Autodesk Fusion 360 part; units mm, degrees
(part 10 of 11)
  spline S28 degree 5 poles (78.2014, 31.4697) (78.2336, 31.4825) (78.2976, 31.5088) (78.3926, 31.5505) (78.5172, 31.6105) (78.6702, 31.6914) (78.8212, 31.7765) (78.9711, 31.8642) (79.1202, 31.9533) (79.269, 32.0433) (79.4172, 32.1344) (79.5647, 32.2267) (79.7114, 32.3207) (79.8571, 32.4168) (80.0017, 32.5149) (80.1454, 32.6148) (80.2882, 32.7163) (80.4303, 32.8191) (80.5718, 32.923) (80.7127, 33.028) (80.853, 33.134) (80.9927, 33.2412) (81.1316, 33.3495) (81.2699, 33.4591) (81.4075, 33.5698) (81.5445, 33.6817) (81.6808, 33.7946) (81.8165, 33.9086) (81.9516, 34.0235) (82.0861, 34.1394) (82.22, 34.2562) (82.3534, 34.374) (82.4862, 34.4927) (82.6183, 34.6123) (82.7499, 34.7329) (82.8809, 34.8543) (83.0114, 34.9766) (83.1413, 35.0998) (83.2706, 35.2239) (83.3993, 35.3487) (83.5276, 35.4744) (83.6552, 35.6009) (83.7824, 35.7282) (83.909, 35.8563) (84.035, 35.9852) (84.1605, 36.1148) (84.2855, 36.2452) (84.4099, 36.3764) (84.5338, 36.5083) (84.6572, 36.641) (84.78, 36.7743) (84.9023, 36.9084) (85.0241, 37.0433) (85.1454, 37.1788) (85.2662, 37.315) (85.3864, 37.4519) (85.5062, 37.5895) (85.6254, 37.7277) (85.7441, 37.8667) (85.8623, 38.0063) (85.9799, 38.1465) (86.0971, 38.2874) (86.2138, 38.429) (86.3299, 38.5712) (86.4456, 38.714) (86.5607, 38.8574) (86.6754, 39.0015) (86.7895, 39.1462) (86.9032, 39.2915) (87.0163, 39.4374) (87.1289, 39.5839) (87.2186, 39.7016) (87.2857, 39.7901) (87.3303, 39.8493) (87.3526, 39.8789) knots 0 0 0 0 0 0 0.01428571 0.02857143 0.04285714 0.05714286 0.07142857 0.08571429 0.1 0.11428571 0.12857143 0.14285714 0.15714286 0.17142857 0.18571429 0.2 0.21428571 0.22857143 0.24285714 0.25714286 0.27142857 0.28571429 0.3 0.31428571 0.32857143 0.34285714 0.35714286 0.37142857 0.38571429 0.4 0.41428571 0.42857143 0.44285714 0.45714286 0.47142857 0.48571429 0.5 0.51428571 0.52857143 0.54285714 0.55714286 0.57142857 0.58571429 0.6 0.61428571 0.62857143 0.64285714 0.65714286 0.67142857 0.68571429 0.7 0.71428571 0.72857143 0.74285714 0.75714286 0.77142857 0.78571429 0.8 0.81428571 0.82857143 0.84285714 0.85714286 0.87142857 0.88571429 0.9 0.91428571 0.92857143 0.94285714 0.95714286 0.97142857 0.98571429 1 1 1 1 1 1
  arc A62 (87.3526, 39.8789) -> (85.3387, 44.0607) centre (0.5538, 0.6546) ccw
  spline S29 degree 5 poles (73.0585, 42.1491) (73.0885, 42.1663) (73.149, 42.1999) (73.2409, 42.2481) (73.3654, 42.3082) (73.5241, 42.3774) (73.6848, 42.4424) (73.8468, 42.5049) (74.0095, 42.5659) (74.1726, 42.6261) (74.3362, 42.6852) (74.5003, 42.743) (74.6653, 42.799) (74.8313, 42.853) (74.9981, 42.9049) (75.1658, 42.955) (75.3342, 43.0033) (75.5032, 43.0504) (75.6727, 43.0962) (75.8426, 43.1409) (76.013, 43.1845) (76.1838, 43.2269) (76.3552, 43.268) (76.527, 43.3078) (76.6994, 43.3463) (76.8722, 43.3837) (77.0455, 43.4198) (77.2192, 43.4548) (77.3933, 43.4888) (77.5678, 43.5217) (77.7426, 43.5536) (77.9179, 43.5844) (78.0934, 43.6142) (78.2694, 43.643) (78.4457, 43.6707) (78.6223, 43.6974) (78.7993, 43.7231) (78.9766, 43.7478) (79.1542, 43.7716) (79.3321, 43.7945) (79.5103, 43.8163) (79.6888, 43.8373) (79.8676, 43.8573) (80.0467, 43.8764) (80.226, 43.8946) (80.4056, 43.9119) (80.5855, 43.9283) (80.7656, 43.9438) (80.946, 43.9584) (81.1267, 43.9722) (81.3075, 43.985) (81.4886, 43.9971) (81.67, 44.0083) (81.8515, 44.0186) (82.0333, 44.0281) (82.2153, 44.0367) (82.3976, 44.0445) (82.58, 44.0515) (82.7626, 44.0577) (82.9454, 44.0631) (83.1285, 44.0677) (83.3117, 44.0714) (83.4951, 44.0744) (83.6787, 44.0765) (83.8625, 44.0779) (84.0464, 44.0785) (84.2305, 44.0783) (84.4148, 44.0773) (84.5993, 44.0756) (84.7839, 44.0731) (84.9686, 44.0698) (85.1166, 44.0665) (85.2276, 44.0638) (85.3017, 44.0618) (85.3387, 44.0607) knots 0 0 0 0 0 0 0.01428571 0.02857143 0.04285714 0.05714286 0.07142857 0.08571429 0.1 0.11428571 0.12857143 0.14285714 0.15714286 0.17142857 0.18571429 0.2 0.21428571 0.22857143 0.24285714 0.25714286 0.27142857 0.28571429 0.3 0.31428571 0.32857143 0.34285714 0.35714286 0.37142857 0.38571429 0.4 0.41428571 0.42857143 0.44285714 0.45714286 0.47142857 0.48571429 0.5 0.51428571 0.52857143 0.54285714 0.55714286 0.57142857 0.58571429 0.6 0.61428571 0.62857143 0.64285714 0.65714286 0.67142857 0.68571429 0.7 0.71428571 0.72857143 0.74285714 0.75714286 0.77142857 0.78571429 0.8 0.81428571 0.82857143 0.84285714 0.85714286 0.87142857 0.88571429 0.9 0.91428571 0.92857143 0.94285714 0.95714286 0.97142857 0.98571429 1 1 1 1 1 1
  line L29 (73.0585, 42.1491) -> (71.7614, 41.4071)
  arc A63 (70.6822, 41.6951) -> (71.7614, 41.4071) centre (71.3673, 42.096) ccw
  arc A64 (70.6822, 41.6951) -> (67.9576, 46.0313) centre (0.5538, 0.6546) ccw
  arc A65 (68.1663, 47.1287) -> (67.9576, 46.0313) centre (68.616, 46.4746) ccw
  line L30 (68.1663, 47.1287) -> (69.3976, 47.9753)
  spline S30 degree 5 poles (69.3976, 47.9753) (69.4262, 47.9949) (69.4827, 48.0348) (69.566, 48.0966) (69.6741, 48.1828) (69.8053, 48.2957) (69.9336, 48.4123) (70.0602, 48.5312) (70.1858, 48.6512) (70.3108, 48.7721) (70.435, 48.8938) (70.5583, 49.0167) (70.6804, 49.141) (70.801, 49.2671) (70.9202, 49.3949) (71.038, 49.5243) (71.1547, 49.655) (71.2704, 49.7869) (71.3852, 49.9197) (71.4992, 50.0534) (71.6124, 50.1879) (71.7247, 50.3235) (71.8361, 50.46) (71.9465, 50.5976) (72.0561, 50.7362) (72.1647, 50.8757) (72.2724, 51.0162) (72.3794, 51.1575) (72.4855, 51.2996) (72.5909, 51.4425) (72.6954, 51.5862) (72.7992, 51.7307) (72.9023, 51.8759) (73.0045, 52.022) (73.106, 52.1688) (73.2067, 52.3164) (73.3066, 52.4646) (73.4058, 52.6136) (73.5043, 52.7633) (73.6021, 52.9137) (73.6991, 53.0648) (73.7954, 53.2165) (73.8911, 53.3689) (73.986, 53.522) (74.0802, 53.6757) (74.1737, 53.83) (74.2665, 53.9849) (74.3586, 54.1405) (74.45, 54.2967) (74.5408, 54.4535) (74.6309, 54.6108) (74.7203, 54.7688) (74.8091, 54.9273) (74.8972, 55.0864) (74.9846, 55.2461) (75.0713, 55.4063) (75.1575, 55.5671) (75.2429, 55.7284) (75.3277, 55.8903) (75.4119, 56.0527) (75.4954, 56.2156) (75.5783, 56.3791) (75.6605, 56.543) (75.7421, 56.7075) (75.8231, 56.8725) (75.9034, 57.0379) (75.9831, 57.2039) (76.0622, 57.3704) (76.1407, 57.5373) (76.2185, 57.7047) (76.2957, 57.8726) (76.357, 58.0073) (76.4027, 58.1086) (76.433, 58.1761) (76.4482, 58.21) knots 0 0 0 0 0 0 0.01428571 0.02857143 0.04285714 0.05714286 0.07142857 0.08571429 0.1 0.11428571 0.12857143 0.14285714 0.15714286 0.17142857 0.18571429 0.2 0.21428571 0.22857143 0.24285714 0.25714286 0.27142857 0.28571429 0.3 0.31428571 0.32857143 0.34285714 0.35714286 0.37142857 0.38571429 0.4 0.41428571 0.42857143 0.44285714 0.45714286 0.47142857 0.48571429 0.5 0.51428571 0.52857143 0.54285714 0.55714286 0.57142857 0.58571429 0.6 0.61428571 0.62857143 0.64285714 0.65714286 0.67142857 0.68571429 0.7 0.71428571 0.72857143 0.74285714 0.75714286 0.77142857 0.78571429 0.8 0.81428571 0.82857143 0.84285714 0.85714286 0.87142857 0.88571429 0.9 0.91428571 0.92857143 0.94285714 0.95714286 0.97142857 0.98571429 1 1 1 1 1 1
  arc A66 (76.4482, 58.21) -> (73.5542, 61.8389) centre (0.5538, 0.6546) ccw
  spline S31 degree 5 poles (62.0072, 57.2425) (62.0327, 57.266) (62.0842, 57.3122) (62.163, 57.3797) (62.2711, 57.4659) (62.4104, 57.5687) (62.5526, 57.6679) (62.6966, 57.7648) (62.8416, 57.8605) (62.9873, 57.9555) (63.1336, 58.0495) (63.2808, 58.1424) (63.4292, 58.2337) (63.579, 58.3233) (63.7301, 58.411) (63.8824, 58.4971) (64.0358, 58.5818) (64.1901, 58.6652) (64.3452, 58.7476) (64.5009, 58.829) (64.6573, 58.9094) (64.8144, 58.9887) (64.9723, 59.067) (65.131, 59.144) (65.2905, 59.22) (65.4507, 59.2948) (65.6116, 59.3686) (65.7731, 59.4414) (65.9353, 59.5133) (66.0981, 59.5842) (66.2614, 59.6542) (66.4254, 59.7232) (66.5899, 59.7913) (66.7551, 59.8585) (66.9208, 59.9248) (67.0871, 59.9901) (67.2539, 60.0545) (67.4212, 60.1181) (67.5891, 60.1808) (67.7575, 60.2427) (67.9263, 60.3037) (68.0957, 60.3638) (68.2655, 60.4231) (68.4359, 60.4816) (68.6067, 60.5392) (68.7779, 60.596) (68.9497, 60.652) (69.1218, 60.7072) (69.2944, 60.7616) (69.4675, 60.8152) (69.6409, 60.8681) (69.8148, 60.9201) (69.9891, 60.9713) (70.1639, 61.0218) (70.339, 61.0715) (70.5145, 61.1204) (70.6904, 61.1686) (70.8667, 61.216) (71.0434, 61.2627) (71.2204, 61.3086) (71.3978, 61.3538) (71.5756, 61.3982) (71.7538, 61.4419) (71.9323, 61.4849) (72.1112, 61.5271) (72.2904, 61.5686) (72.4699, 61.6094) (72.6498, 61.6494) (72.83, 61.6888) (73.0105, 61.7274) (73.1914, 61.7653) (73.3364, 61.7951) (73.4452, 61.8171) (73.5179, 61.8316) (73.5542, 61.8389) knots 0 0 0 0 0 0 0.01428571 0.02857143 0.04285714 0.05714286 0.07142857 0.08571429 0.1 0.11428571 0.12857143 0.14285714 0.15714286 0.17142857 0.18571429 0.2 0.21428571 0.22857143 0.24285714 0.25714286 0.27142857 0.28571429 0.3 0.31428571 0.32857143 0.34285714 0.35714286 0.37142857 0.38571429 0.4 0.41428571 0.42857143 0.44285714 0.45714286 0.47142857 0.48571429 0.5 0.51428571 0.52857143 0.54285714 0.55714286 0.57142857 0.58571429 0.6 0.61428571 0.62857143 0.64285714 0.65714286 0.67142857 0.68571429 0.7 0.71428571 0.72857143 0.74285714 0.75714286 0.77142857 0.78571429 0.8 0.81428571 0.82857143 0.84285714 0.85714286 0.87142857 0.88571429 0.9 0.91428571 0.92857143 0.94285714 0.95714286 0.97142857 0.98571429 1 1 1 1 1 1
  line L31 (62.0072, 57.2425) -> (60.9079, 56.2305)
  arc A67 (59.7916, 56.2712) -> (60.9079, 56.2305) centre (60.3703, 56.8145) ccw
  arc A68 (59.7916, 56.2712) -> (56.1704, 59.8924) centre (0.5538, 0.6546) ccw
  arc A69 (56.1297, 61.0086) -> (56.1704, 59.8924) centre (56.7137, 60.4711) ccw
  line L32 (56.1297, 61.0086) -> (57.1417, 62.108)
  spline S32 degree 5 poles (57.1417, 62.108) (57.1652, 62.1335) (57.2114, 62.185) (57.2789, 62.2638) (57.3651, 62.3719) (57.4679, 62.5112) (57.5671, 62.6534) (57.664, 62.7974) (57.7597, 62.9424) (57.8547, 63.0881) (57.9487, 63.2344) (58.0416, 63.3816) (58.1329, 63.53) (58.2225, 63.6797) (58.3102, 63.8309) (58.3963, 63.9832) (58.481, 64.1366) (58.5644, 64.2909) (58.6468, 64.4459) (58.7282, 64.6017) (58.8086, 64.7581) (58.8879, 64.9152) (58.9662, 65.0731) (59.0432, 65.2318) (59.1192, 65.3913) (59.194, 65.5515) (59.2678, 65.7124) (59.3406, 65.8739) (59.4125, 66.0361) (59.4834, 66.1989) (59.5534, 66.3622) (59.6224, 66.5262) (59.6905, 66.6907) (59.7577, 66.8559) (59.824, 67.0216) (59.8893, 67.1879) (59.9537, 67.3547) (60.0173, 67.522) (60.08, 67.6899) (60.1419, 67.8583) (60.2029, 68.0271) (60.263, 68.1965) (60.3223, 68.3663) (60.3808, 68.5367) (60.4384, 68.7075) (60.4952, 68.8787) (60.5512, 69.0505) (60.6064, 69.2226) (60.6608, 69.3952) (60.7144, 69.5683) (60.7673, 69.7417) (60.8193, 69.9156) (60.8705, 70.0899) (60.921, 70.2647) (60.9707, 70.4398) (61.0196, 70.6153) (61.0678, 70.7912) (61.1152, 70.9675) (61.1619, 71.1442) (61.2078, 71.3212) (61.253, 71.4986) (61.2974, 71.6764) (61.3411, 71.8546) (61.3841, 72.0331) (61.4263, 72.212) (61.4678, 72.3912) (61.5086, 72.5707) (61.5486, 72.7506) (61.588, 72.9308) (61.6266, 73.1113) (61.6645, 73.2922) (61.6943, 73.4372) (61.7163, 73.546) (61.7308, 73.6187) (61.7381, 73.655) knots 0 0 0 0 0 0 0.01428571 0.02857143 0.04285714 0.05714286 0.07142857 0.08571429 0.1 0.11428571 0.12857143 0.14285714 0.15714286 0.17142857 0.18571429 0.2 0.21428571 0.22857143 0.24285714 0.25714286 0.27142857 0.28571429 0.3 0.31428571 0.32857143 0.34285714 0.35714286 0.37142857 0.38571429 0.4 0.41428571 0.42857143 0.44285714 0.45714286 0.47142857 0.48571429 0.5 0.51428571 0.52857143 0.54285714 0.55714286 0.57142857 0.58571429 0.6 0.61428571 0.62857143 0.64285714 0.65714286 0.67142857 0.68571429 0.7 0.71428571 0.72857143 0.74285714 0.75714286 0.77142857 0.78571429 0.8 0.81428571 0.82857143 0.84285714 0.85714286 0.87142857 0.88571429 0.9 0.91428571 0.92857143 0.94285714 0.95714286 0.97142857 0.98571429 1 1 1 1 1 1
  arc A70 (61.7381, 73.655) -> (58.1092, 76.549) centre (0.5538, 0.6546) ccw
  spline S33 degree 5 poles (47.8745, 69.4984) (47.8941, 69.527) (47.934, 69.5835) (47.9958, 69.6668) (48.082, 69.7749) (48.1949, 69.9061) (48.3115, 70.0344) (48.4304, 70.161) (48.5504, 70.2866) (48.6713, 70.4116) (48.793, 70.5358) (48.9159, 70.6591) (49.0402, 70.7812) (49.1663, 70.9018) (49.2941, 71.021) (49.4235, 71.1388) (49.5542, 71.2555) (49.6861, 71.3712) (49.8189, 71.486) (49.9526, 71.6) (50.0871, 71.7132) (50.2227, 71.8255) (50.3592, 71.9369) (50.4968, 72.0473) (50.6354, 72.1569) (50.7749, 72.2655) (50.9154, 72.3732) (51.0567, 72.4802) (51.1988, 72.5863) (51.3417, 72.6917) (51.4854, 72.7962) (51.6299, 72.9) (51.7751, 73.0031) (51.9212, 73.1053) (52.068, 73.2068) (52.2156, 73.3075) (52.3638, 73.4074) (52.5129, 73.5066) (52.6626, 73.6051) (52.8129, 73.7029) (52.964, 73.7999) (53.1157, 73.8962) (53.2681, 73.9919) (53.4212, 74.0868) (53.5749, 74.181) (53.7292, 74.2745) (53.8842, 74.3673) (54.0397, 74.4594) (54.1959, 74.5508) (54.3527, 74.6416) (54.51, 74.7317) (54.668, 74.8211) (54.8265, 74.9099) (54.9856, 74.998) (55.1453, 75.0854) (55.3055, 75.1721) (55.4663, 75.2583) (55.6276, 75.3437) (55.7895, 75.4285) (55.9519, 75.5127) (56.1148, 75.5962) (56.2783, 75.6791) (56.4422, 75.7613) (56.6067, 75.8429) (56.7717, 75.9239) (56.9371, 76.0042) (57.1031, 76.0839) (57.2696, 76.163) (57.4365, 76.2415) (57.6039, 76.3193) (57.7718, 76.3965) (57.9065, 76.4578) (58.0078, 76.5035) (58.0753, 76.5338) (58.1092, 76.549) knots 0 0 0 0 0 0 0.01428571 0.02857143 0.04285714 0.05714286 0.07142857 0.08571429 0.1 0.11428571 0.12857143 0.14285714 0.15714286 0.17142857 0.18571429 0.2 0.21428571 0.22857143 0.24285714 0.25714286 0.27142857 0.28571429 0.3 0.31428571 0.32857143 0.34285714 0.35714286 0.37142857 0.38571429 0.4 0.41428571 0.42857143 0.44285714 0.45714286 0.47142857 0.48571429 0.5 0.51428571 0.52857143 0.54285714 0.55714286 0.57142857 0.58571429 0.6 0.61428571 0.62857143 0.64285714 0.65714286 0.67142857 0.68571429 0.7 0.71428571 0.72857143 0.74285714 0.75714286 0.77142857 0.78571429 0.8 0.81428571 0.82857143 0.84285714 0.85714286 0.87142857 0.88571429 0.9 0.91428571 0.92857143 0.94285714 0.95714286 0.97142857 0.98571429 1 1 1 1 1 1
  line L33 (47.8745, 69.4984) -> (47.0279, 68.2671)
  arc A71 (45.9305, 68.0584) -> (47.0279, 68.2671) centre (46.3738, 68.7168) ccw
  arc A72 (45.9305, 68.0584) -> (41.5943, 70.783) centre (0.5538, 0.6546) ccw
  arc A73 (41.3063, 71.8622) -> (41.5943, 70.783) centre (41.9952, 71.4681) ccw
  line L34 (41.3063, 71.8622) -> (42.0483, 73.1593)
  spline S34 degree 5 poles (42.0483, 73.1593) (42.0655, 73.1893) (42.0991, 73.2498) (42.1473, 73.3417) (42.2074, 73.4662) (42.2766, 73.6249) (42.3416, 73.7856) (42.4041, 73.9476) (42.4651, 74.1103) (42.5253, 74.2734) (42.5844, 74.437) (42.6422, 74.6011) (42.6982, 74.7661) (42.7522, 74.9321) (42.8041, 75.0989) (42.8542, 75.2666) (42.9025, 75.435) (42.9496, 75.604) (42.9954, 75.7735) (43.0401, 75.9434) (43.0837, 76.1138) (43.1261, 76.2846) (43.1672, 76.456) (43.207, 76.6278) (43.2456, 76.8002) (43.2829, 76.973) (43.319, 77.1463) (43.354, 77.32) (43.388, 77.4941) (43.4209, 77.6686) (43.4528, 77.8434) (43.4836, 78.0187) (43.5134, 78.1942) (43.5422, 78.3702) (43.5699, 78.5465) (43.5966, 78.7231) (43.6223, 78.9001) (43.6471, 79.0774) (43.6708, 79.255) (43.6937, 79.4329) (43.7155, 79.6111) (43.7365, 79.7896) (43.7565, 79.9684) (43.7756, 80.1475) (43.7938, 80.3268) (43.8111, 80.5064) (43.8275, 80.6863) (43.843, 80.8664) (43.8576, 81.0468) (43.8714, 81.2275) (43.8842, 81.4083) (43.8963, 81.5894) (43.9075, 81.7708) (43.9178, 81.9523) (43.9273, 82.1341) (43.9359, 82.3161) (43.9437, 82.4984) (43.9507, 82.6808) (43.9569, 82.8634) (43.9623, 83.0462) (43.9669, 83.2293) (43.9706, 83.4125) (43.9736, 83.5959) (43.9757, 83.7795) (43.9771, 83.9633) (43.9777, 84.1472) (43.9775, 84.3313) (43.9765, 84.5156) (43.9748, 84.7001) (43.9723, 84.8847) (43.969, 85.0694) (43.9657, 85.2174) (43.963, 85.3284) (43.961, 85.4025) (43.9599, 85.4395) knots 0 0 0 0 0 0 0.01428571 0.02857143 0.04285714 0.05714286 0.07142857 0.08571429 0.1 0.11428571 0.12857143 0.14285714 0.15714286 0.17142857 0.18571429 0.2 0.21428571 0.22857143 0.24285714 0.25714286 0.27142857 0.28571429 0.3 0.31428571 0.32857143 0.34285714 0.35714286 0.37142857 0.38571429 0.4 0.41428571 0.42857143 0.44285714 0.45714286 0.47142857 0.48571429 0.5 0.51428571 0.52857143 0.54285714 0.55714286 0.57142857 0.58571429 0.6 0.61428571 0.62857143 0.64285714 0.65714286 0.67142857 0.68571429 0.7 0.71428571 0.72857143 0.74285714 0.75714286 0.77142857 0.78571429 0.8 0.81428571 0.82857143 0.84285714 0.85714286 0.87142857 0.88571429 0.9 0.91428571 0.92857143 0.94285714 0.95714286 0.97142857 0.98571429 1 1 1 1 1 1
  arc A74 (43.9599, 85.4395) -> (39.7781, 87.4534) centre (0.5538, 0.6546) ccw
  spline S35 degree 5 poles (31.3689, 78.3022) (31.3817, 78.3344) (31.408, 78.3984) (31.4497, 78.4934) (31.5097, 78.618) (31.5906, 78.771) (31.6757, 78.922) (31.7634, 79.0719) (31.8525, 79.221) (31.9425, 79.3697) (32.0336, 79.518) (32.1259, 79.6655) (32.2199, 79.8122) (32.316, 79.9579) (32.4141, 80.1025) (32.514, 80.2462) (32.6155, 80.389) (32.7183, 80.5311) (32.8222, 80.6726) (32.9272, 80.8135) (33.0332, 80.9538) (33.1404, 81.0935) (33.2487, 81.2324) (33.3583, 81.3707) (33.469, 81.5083) (33.5809, 81.6453) (33.6938, 81.7816) (33.8078, 81.9173) (33.9227, 82.0524) (34.0386, 82.1869) (34.1554, 82.3208) (34.2732, 82.4542) (34.3919, 82.587) (34.5115, 82.7191) (34.6321, 82.8507) (34.7535, 82.9817) (34.8758, 83.1122) (34.999, 83.242) (35.1231, 83.3714) (35.2479, 83.5001) (35.3736, 83.6284) (35.5001, 83.756) (35.6274, 83.8832) (35.7555, 84.0098) (35.8844, 84.1358) (36.014, 84.2613) (36.1444, 84.3863) (36.2756, 84.5107) (36.4075, 84.6346) (36.5402, 84.758) (36.6735, 84.8808) (36.8076, 85.0031) (36.9425, 85.1249) (37.078, 85.2462) (37.2142, 85.367) (37.3511, 85.4872) (37.4887, 85.607) (37.6269, 85.7262) (37.7659, 85.8449) (37.9055, 85.9631) (38.0457, 86.0807) (38.1866, 86.1979) (38.3282, 86.3146) (38.4704, 86.4307) (38.6132, 86.5464) (38.7566, 86.6615) (38.9007, 86.7762) (39.0454, 86.8903) (39.1907, 87.0039) (39.3366, 87.1171) (39.4831, 87.2297) (39.6008, 87.3194) (39.6893, 87.3865) (39.7485, 87.4311) (39.7781, 87.4534) knots 0 0 0 0 0 0 0.01428571 0.02857143 0.04285714 0.05714286 0.07142857 0.08571429 0.1 0.11428571 0.12857143 0.14285714 0.15714286 0.17142857 0.18571429 0.2 0.21428571 0.22857143 0.24285714 0.25714286 0.27142857 0.28571429 0.3 0.31428571 0.32857143 0.34285714 0.35714286 0.37142857 0.38571429 0.4 0.41428571 0.42857143 0.44285714 0.45714286 0.47142857 0.48571429 0.5 0.51428571 0.52857143 0.54285714 0.55714286 0.57142857 0.58571429 0.6 0.61428571 0.62857143 0.64285714 0.65714286 0.67142857 0.68571429 0.7 0.71428571 0.72857143 0.74285714 0.75714286 0.77142857 0.78571429 0.8 0.81428571 0.82857143 0.84285714 0.85714286 0.87142857 0.88571429 0.9 0.91428571 0.92857143 0.94285714 0.95714286 0.97142857 0.98571429 1 1 1 1 1 1
  line L35 (31.3689, 78.3022) -> (30.8175, 76.9134)
  arc A75 (29.7941, 76.4657) -> (30.8175, 76.9134) centre (30.0797, 77.2063) ccw
  arc A76 (29.7941, 76.4657) -> (24.9603, 78.1571) centre (0.5538, 0.6546) ccw
  arc A77 (24.4393, 79.1452) -> (24.9603, 78.1571) centre (25.1987, 78.9142) ccw
  line L36 (24.4393, 79.1452) -> (24.8741, 80.5748)
  spline S36 degree 5 poles (24.8741, 80.5748) (24.8842, 80.6079) (24.9035, 80.6744) (24.9301, 80.7747) (24.9609, 80.9095) (24.9931, 81.0795) (25.0207, 81.2507) (25.0456, 81.4225) (25.0689, 81.5947) (25.0912, 81.7671) (25.1125, 81.9398) (25.1323, 82.1127) (25.1502, 82.286) (25.1659, 82.4598) (25.1794, 82.634) (25.1909, 82.8086) (25.2006, 82.9836) (25.2088, 83.1588) (25.2158, 83.3342) (25.2216, 83.5098) (25.2261, 83.6856) (25.2294, 83.8616) (25.2314, 84.0378) (25.232, 84.2142) (25.2312, 84.3909) (25.2291, 84.5677) (25.2258, 84.7447) (25.2213, 84.9218) (25.2157, 85.0991) (25.209, 85.2765) (25.2011, 85.4541) (25.1922, 85.6318) (25.1822, 85.8096) (25.171, 85.9875) (25.1588, 86.1655) (25.1456, 86.3437) (25.1312, 86.522) (25.1159, 86.7003) (25.0996, 86.8787) (25.0822, 87.0573) (25.0639, 87.2359) (25.0446, 87.4146) (25.0244, 87.5933) (25.0031, 87.7722) (24.981, 87.9511) (24.9578, 88.13) (24.9338, 88.309) (24.9088, 88.4881) (24.8829, 88.6672) (24.8562, 88.8464) (24.8285, 89.0256) (24.7999, 89.2048) (24.7705, 89.3841) (24.7401, 89.5634) (24.7089, 89.7428) (24.6769, 89.9221) (24.6439, 90.1015) (24.6102, 90.2809) (24.5755, 90.4604) (24.5401, 90.6398) (24.5038, 90.8193) (24.4667, 90.9987) (24.4288, 91.1782) (24.39, 91.3576) (24.3505, 91.5371) (24.3101, 91.7166) (24.2689, 91.896) (24.227, 92.0755) (24.1843, 92.2549) (24.1407, 92.4344) (24.0964, 92.6138) (24.0603, 92.7573) (24.0329, 92.8649) (24.0145, 92.9367) (24.0053, 92.9725) knots 0 0 0 0 0 0 0.01428571 0.02857143 0.04285714 0.05714286 0.07142857 0.08571429 0.1 0.11428571 0.12857143 0.14285714 0.15714286 0.17142857 0.18571429 0.2 0.21428571 0.22857143 0.24285714 0.25714286 0.27142857 0.28571429 0.3 0.31428571 0.32857143 0.34285714 0.35714286 0.37142857 0.38571429 0.4 0.41428571 0.42857143 0.44285714 0.45714286 0.47142857 0.48571429 0.5 0.51428571 0.52857143 0.54285714 0.55714286 0.57142857 0.58571429 0.6 0.61428571 0.62857143 0.64285714 0.65714286 0.67142857 0.68571429 0.7 0.71428571 0.72857143 0.74285714 0.75714286 0.77142857 0.78571429 0.8 0.81428571 0.82857143 0.84285714 0.85714286 0.87142857 0.88571429 0.9 0.91428571 0.92857143 0.94285714 0.95714286 0.97142857 0.98571429 1 1 1 1 1 1
  arc A78 (24.0053, 92.9725) -> (19.4801, 94.0054) centre (0.5538, 0.6546) ccw
  spline S37 degree 5 poles (13.3181, 83.2124) (13.3234, 83.2466) (13.3348, 83.3149) (13.3544, 83.4168) (13.3851, 83.5516) (13.4299, 83.7188) (13.4793, 83.8849) (13.5314, 84.0505) (13.5851, 84.2158) (13.6398, 84.3808) (13.6955, 84.5456) (13.7527, 84.71) (13.8118, 84.8739) (13.873, 85.0373) (13.9365, 85.2001) (14.0019, 85.3624) (14.0691, 85.5243) (14.1377, 85.6857) (14.2075, 85.8468) (14.2785, 86.0075) (14.3507, 86.1679) (14.424, 86.3279) (14.4987, 86.4875) (14.5748, 86.6467) (14.6521, 86.8055) (14.7307, 86.9639) (14.8105, 87.1219) (14.8914, 87.2796) (14.9734, 87.4368) (15.0564, 87.5938) (15.1405, 87.7503) (15.2256, 87.9066) (15.3118, 88.0624) (15.399, 88.2179) (15.4873, 88.373) (15.5766, 88.5278) (15.6668, 88.6822) (15.758, 88.8362) (15.8501, 88.9899) (15.9432, 89.1432) (16.0372, 89.2962) (16.1321, 89.4488) (16.2279, 89.6011) (16.3247, 89.753) (16.4223, 89.9045) (16.5207, 90.0557) (16.6201, 90.2066) (16.7203, 90.3571) (16.8213, 90.5072) (16.9232, 90.657) (17.0259, 90.8065) (17.1294, 90.9556) (17.2337, 91.1043) (17.3388, 91.2527) (17.4448, 91.4008) (17.5515, 91.5485) (17.659, 91.6958) (17.7672, 91.8428) (17.8763, 91.9894) (17.9861, 92.1357) (18.0966, 92.2817) (18.2079, 92.4272) (18.32, 92.5725) (18.4327, 92.7174) (18.5462, 92.8619) (18.6605, 93.0061) (18.7754, 93.1499) (18.8911, 93.2934) (19.0075, 93.4365) (19.1245, 93.5793) (19.2423, 93.7217) (19.3371, 93.8353) (19.4084, 93.9204) (19.4562, 93.9771) (19.4801, 94.0054) knots 0 0 0 0 0 0 0.01428571 0.02857143 0.04285714 0.05714286 0.07142857 0.08571429 0.1 0.11428571 0.12857143 0.14285714 0.15714286 0.17142857 0.18571429 0.2 0.21428571 0.22857143 0.24285714 0.25714286 0.27142857 0.28571429 0.3 0.31428571 0.32857143 0.34285714 0.35714286 0.37142857 0.38571429 0.4 0.41428571 0.42857143 0.44285714 0.45714286 0.47142857 0.48571429 0.5 0.51428571 0.52857143 0.54285714 0.55714286 0.57142857 0.58571429 0.6 0.61428571 0.62857143 0.64285714 0.65714286 0.67142857 0.68571429 0.7 0.71428571 0.72857143 0.74285714 0.75714286 0.77142857 0.78571429 0.8 0.81428571 0.82857143 0.84285714 0.85714286 0.87142857 0.88571429 0.9 0.91428571 0.92857143 0.94285714 0.95714286 0.97142857 0.98571429 1 1 1 1 1 1
  line L37 (13.3181, 83.2124) -> (13.0895, 81.7357)
  arc A79 (12.1914, 81.0715) -> (13.0895, 81.7357) centre (12.3051, 81.8571) ccw
  arc A80 (12.1914, 81.0715) -> (7.1025, 81.6449) centre (0.5538, 0.6546) ccw
  arc A81 (6.3747, 82.4923) -> (7.1025, 81.6449) centre (7.1664, 82.4361) ccw
  line L38 (6.3747, 82.4923) -> (6.4805, 83.9828)
  spline S38 degree 5 poles (6.4805, 83.9828) (6.4829, 84.0174) (6.487, 84.0864) (6.4906, 84.1901) (6.4906, 84.3284) (6.4841, 84.5014) (6.473, 84.6744) (6.459, 84.8474) (6.4434, 85.0205) (6.4268, 85.1935) (6.4091, 85.3666) (6.39, 85.5396) (6.3689, 85.7126) (6.3455, 85.8855) (6.3199, 86.0583) (6.2922, 86.2311) (6.2627, 86.4038) (6.2318, 86.5765) (6.1995, 86.7491) (6.1661, 86.9216) (6.1314, 87.094) (6.0955, 87.2663) (6.0582, 87.4385) (6.0195, 87.6106) (5.9794, 87.7827) (5.9381, 87.9546) (5.8954, 88.1264) (5.8516, 88.2981) (5.8067, 88.4697) (5.7607, 88.6412) (5.7135, 88.8125) (5.6653, 88.9838) (5.6159, 89.1549) (5.5655, 89.3259) (5.514, 89.4967) (5.4614, 89.6675) (5.4078, 89.8381) (5.3531, 90.0085) (5.2975, 90.1789) (5.2409, 90.3491) (5.1833, 90.5191) (5.1247, 90.689) (5.0652, 90.8588) (5.0047, 91.0284) (4.9432, 91.1979) (4.8809, 91.3672) (4.8176, 91.5364) (4.7534, 91.7054) (4.6883, 91.8743) (4.6223, 92.043) (4.5555, 92.2116) (4.4877, 92.38) (4.4191, 92.5482) (4.3497, 92.7162) (4.2793, 92.8842) (4.2082, 93.0519) (4.1361, 93.2195) (4.0633, 93.3869) (3.9896, 93.5541) (3.9151, 93.7211) (3.8398, 93.888) (3.7637, 94.0547) (3.6868, 94.2212) (3.6091, 94.3876) (3.5306, 94.5538) (3.4513, 94.7197) (3.3712, 94.8855) (3.2904, 95.0512) (3.2088, 95.2166) (3.1264, 95.3818) (3.0433, 95.5469) (2.9762, 95.6788) (2.9255, 95.7776) (2.8916, 95.8434) (2.8746, 95.8764) knots 0 0 0 0 0 0 0.01428571 0.02857143 0.04285714 0.05714286 0.07142857 0.08571429 0.1 0.11428571 0.12857143 0.14285714 0.15714286 0.17142857 0.18571429 0.2 0.21428571 0.22857143 0.24285714 0.25714286 0.27142857 0.28571429 0.3 0.31428571 0.32857143 0.34285714 0.35714286 0.37142857 0.38571429 0.4 0.41428571 0.42857143 0.44285714 0.45714286 0.47142857 0.48571429 0.5 0.51428571 0.52857143 0.54285714 0.55714286 0.57142857 0.58571429 0.6 0.61428571 0.62857143 0.64285714 0.65714286 0.67142857 0.68571429 0.7 0.71428571 0.72857143 0.74285714 0.75714286 0.77142857 0.78571429 0.8 0.81428571 0.82857143 0.84285714 0.85714286 0.87142857 0.88571429 0.9 0.91428571 0.92857143 0.94285714 0.95714286 0.97142857 0.98571429 1 1 1 1 1 1
  arc A82 (2.8746, 95.8764) -> (-1.7669, 95.8764) centre (0.5538, 0.6546) ccw
  spline S39 degree 5 poles (-5.3728, 83.9828) (-5.3752, 84.0174) (-5.3793, 84.0864) (-5.3829, 84.1901) (-5.3829, 84.3284) (-5.3764, 84.5014) (-5.3653, 84.6744) (-5.3513, 84.8474) (-5.3357, 85.0205) (-5.3191, 85.1935) (-5.3014, 85.3666) (-5.2823, 85.5396) (-5.2612, 85.7126) (-5.2378, 85.8855) (-5.2122, 86.0583) (-5.1845, 86.2311) (-5.155, 86.4038) (-5.1241, 86.5765) (-5.0918, 86.7491) (-5.0584, 86.9216) (-5.0237, 87.094) (-4.9878, 87.2663) (-4.9505, 87.4385) (-4.9118, 87.6106) (-4.8717, 87.7827) (-4.8304, 87.9546) (-4.7877, 88.1264) (-4.7439, 88.2981) (-4.699, 88.4697) (-4.653, 88.6412) (-4.6058, 88.8125) (-4.5576, 88.9838) (-4.5082, 89.1549) (-4.4578, 89.3259) (-4.4063, 89.4967) (-4.3537, 89.6675) (-4.3001, 89.8381) (-4.2454, 90.0085) (-4.1898, 90.1789) (-4.1332, 90.3491) (-4.0756, 90.5191) (-4.017, 90.689) (-3.9575, 90.8588) (-3.897, 91.0284) (-3.8356, 91.1979) (-3.7732, 91.3672) (-3.7099, 91.5364) (-3.6457, 91.7054) (-3.5806, 91.8743) (-3.5147, 92.043) (-3.4478, 92.2116) (-3.3801, 92.38) (-3.3114, 92.5482) (-3.242, 92.7162) (-3.1716, 92.8842) (-3.1005, 93.0519) (-3.0285, 93.2195) (-2.9556, 93.3869) (-2.8819, 93.5541) (-2.8074, 93.7211) (-2.7321, 93.888) (-2.656, 94.0547) (-2.5791, 94.2212) (-2.5014, 94.3876) (-2.4229, 94.5538) (-2.3436, 94.7197) (-2.2636, 94.8855) (-2.1827, 95.0512) (-2.1011, 95.2166) (-2.0188, 95.3818) (-1.9356, 95.5469) (-1.8685, 95.6788) (-1.8179, 95.7776) (-1.7839, 95.8434) (-1.7669, 95.8764) knots 0 0 0 0 0 0 0.01428571 0.02857143 0.04285714 0.05714286 0.07142857 0.08571429 0.1 0.11428571 0.12857143 0.14285714 0.15714286 0.17142857 0.18571429 0.2 0.21428571 0.22857143 0.24285714 0.25714286 0.27142857 0.28571429 0.3 0.31428571 0.32857143 0.34285714 0.35714286 0.37142857 0.38571429 0.4 0.41428571 0.42857143 0.44285714 0.45714286 0.47142857 0.48571429 0.5 0.51428571 0.52857143 0.54285714 0.55714286 0.57142857 0.58571429 0.6 0.61428571 0.62857143 0.64285714 0.65714286 0.67142857 0.68571429 0.7 0.71428571 0.72857143 0.74285714 0.75714286 0.77142857 0.78571429 0.8 0.81428571 0.82857143 0.84285714 0.85714286 0.87142857 0.88571429 0.9 0.91428571 0.92857143 0.94285714 0.95714286 0.97142857 0.98571429 1 1 1 1 1 1
  line L39 (-5.3728, 83.9828) -> (-5.267, 82.4923)
  arc A83 (-5.9948, 81.6449) -> (-5.267, 82.4923) centre (-6.0588, 82.4361) ccw
  arc A84 (-5.9948, 81.6449) -> (-11.0838, 81.0715) centre (0.5538, 0.6546) ccw
  arc A85 (-11.9819, 81.7357) -> (-11.0838, 81.0715) centre (-11.1974, 81.8571) ccw
  line L40 (-11.9819, 81.7357) -> (-12.2104, 83.2124)
  spline S40 degree 5 poles (-12.2104, 83.2124) (-12.2157, 83.2466) (-12.2271, 83.3149) (-12.2467, 83.4168) (-12.2774, 83.5516) (-12.3222, 83.7188) (-12.3716, 83.8849) (-12.4237, 84.0505) (-12.4774, 84.2158) (-12.5321, 84.3808) (-12.5879, 84.5456) (-12.645, 84.71) (-12.7041, 84.8739) (-12.7654, 85.0373) (-12.8288, 85.2001) (-12.8942, 85.3624) (-12.9614, 85.5243) (-13.03, 85.6857) (-13.0998, 85.8468) (-13.1708, 86.0075) (-13.243, 86.1679) (-13.3164, 86.3279) (-13.3911, 86.4875) (-13.4671, 86.6467) (-13.5444, 86.8055) (-13.623, 86.9639) (-13.7028, 87.1219) (-13.7837, 87.2796) (-13.8657, 87.4368) (-13.9487, 87.5938) (-14.0328, 87.7503) (-14.118, 87.9066) (-14.2041, 88.0624) (-14.2914, 88.2179) (-14.3796, 88.373) (-14.4689, 88.5278) (-14.5591, 88.6822) (-14.6503, 88.8362) (-14.7425, 88.9899) (-14.8355, 89.1432) (-14.9295, 89.2962) (-15.0244, 89.4488) (-15.1203, 89.6011) (-15.217, 89.753) (-15.3146, 89.9045) (-15.4131, 90.0557) (-15.5124, 90.2066) (-15.6126, 90.3571) (-15.7136, 90.5072) (-15.8155, 90.657) (-15.9182, 90.8065) (-16.0217, 90.9556) (-16.126, 91.1043) (-16.2312, 91.2527) (-16.3371, 91.4008) (-16.4438, 91.5485) (-16.5513, 91.6958) (-16.6596, 91.8428) (-16.7686, 91.9894) (-16.8784, 92.1357) (-16.9889, 92.2817) (-17.1002, 92.4272) (-17.2123, 92.5725) (-17.3251, 92.7174) (-17.4386, 92.8619) (-17.5528, 93.0061) (-17.6677, 93.1499) (-17.7834, 93.2934) (-17.8998, 93.4365) (-18.0168, 93.5793) (-18.1346, 93.7217) (-18.2294, 93.8353) (-18.3008, 93.9204) (-18.3485, 93.9771) (-18.3724, 94.0054) knots 0 0 0 0 0 0 0.01428571 0.02857143 0.04285714 0.05714286 0.07142857 0.08571429 0.1 0.11428571 0.12857143 0.14285714 0.15714286 0.17142857 0.18571429 0.2 0.21428571 0.22857143 0.24285714 0.25714286 0.27142857 0.28571429 0.3 0.31428571 0.32857143 0.34285714 0.35714286 0.37142857 0.38571429 0.4 0.41428571 0.42857143 0.44285714 0.45714286 0.47142857 0.48571429 0.5 0.51428571 0.52857143 0.54285714 0.55714286 0.57142857 0.58571429 0.6 0.61428571 0.62857143 0.64285714 0.65714286 0.67142857 0.68571429 0.7 0.71428571 0.72857143 0.74285714 0.75714286 0.77142857 0.78571429 0.8 0.81428571 0.82857143 0.84285714 0.85714286 0.87142857 0.88571429 0.9 0.91428571 0.92857143 0.94285714 0.95714286 0.97142857 0.98571429 1 1 1 1 1 1
  arc A86 (-18.3724, 94.0054) -> (-22.8976, 92.9725) centre (0.5538, 0.6546) ccw
  spline S41 degree 5 poles (-23.7664, 80.5748) (-23.7765, 80.6079) (-23.7959, 80.6744) (-23.8224, 80.7747) (-23.8532, 80.9095) (-23.8854, 81.0795) (-23.913, 81.2507) (-23.9379, 81.4225) (-23.9612, 81.5947) (-23.9836, 81.7671) (-24.0048, 81.9398) (-24.0246, 82.1127) (-24.0425, 82.286) (-24.0582, 82.4598) (-24.0717, 82.634) (-24.0832, 82.8086) (-24.0929, 82.9836) (-24.1011, 83.1588) (-24.1081, 83.3342) (-24.1139, 83.5098) (-24.1185, 83.6856) (-24.1218, 83.8616) (-24.1237, 84.0378) (-24.1243, 84.2142) (-24.1235, 84.3909) (-24.1214, 84.5677) (-24.1181, 84.7447) (-24.1136, 84.9218) (-24.108, 85.0991) (-24.1013, 85.2765) (-24.0934, 85.4541) (-24.0845, 85.6318) (-24.0745, 85.8096) (-24.0634, 85.9875) (-24.0512, 86.1655) (-24.0379, 86.3437) (-24.0236, 86.522) (-24.0082, 86.7003) (-23.9919, 86.8787) (-23.9746, 87.0573) (-23.9562, 87.2359) (-23.9369, 87.4146) (-23.9167, 87.5933) (-23.8955, 87.7722) (-23.8733, 87.9511) (-23.8502, 88.13) (-23.8261, 88.309) (-23.8011, 88.4881) (-23.7753, 88.6672) (-23.7485, 88.8464) (-23.7208, 89.0256) (-23.6922, 89.2048) (-23.6628, 89.3841) (-23.6324, 89.5634) (-23.6012, 89.7428) (-23.5692, 89.9221) (-23.5362, 90.1015) (-23.5025, 90.2809) (-23.4679, 90.4604) (-23.4324, 90.6398) (-23.3961, 90.8193) (-23.359, 90.9987) (-23.3211, 91.1782) (-23.2823, 91.3576) (-23.2428, 91.5371) (-23.2024, 91.7166) (-23.1613, 91.896) (-23.1193, 92.0755) (-23.0766, 92.2549) (-23.033, 92.4344) (-22.9887, 92.6138) (-22.9527, 92.7573) (-22.9253, 92.8649) (-22.9068, 92.9367) (-22.8976, 92.9725) knots 0 0 0 0 0 0 0.01428571 0.02857143 0.04285714 0.05714286 0.07142857 0.08571429 0.1 0.11428571 0.12857143 0.14285714 0.15714286 0.17142857 0.18571429 0.2 0.21428571 0.22857143 0.24285714 0.25714286 0.27142857 0.28571429 0.3 0.31428571 0.32857143 0.34285714 0.35714286 0.37142857 0.38571429 0.4 0.41428571 0.42857143 0.44285714 0.45714286 0.47142857 0.48571429 0.5 0.51428571 0.52857143 0.54285714 0.55714286 0.57142857 0.58571429 0.6 0.61428571 0.62857143 0.64285714 0.65714286 0.67142857 0.68571429 0.7 0.71428571 0.72857143 0.74285714 0.75714286 0.77142857 0.78571429 0.8 0.81428571 0.82857143 0.84285714 0.85714286 0.87142857 0.88571429 0.9 0.91428571 0.92857143 0.94285714 0.95714286 0.97142857 0.98571429 1 1 1 1 1 1
  line L41 (-23.7664, 80.5748) -> (-23.3316, 79.1452)
  arc A87 (-23.8526, 78.1571) -> (-23.3316, 79.1452) centre (-24.091, 78.9142) ccw
  arc A88 (-23.8526, 78.1571) -> (-28.6864, 76.4657) centre (0.5538, 0.6546) ccw
  arc A89 (-29.7098, 76.9134) -> (-28.6864, 76.4657) centre (-28.9721, 77.2063) ccw
  line L42 (-29.7098, 76.9134) -> (-30.2612, 78.3022)
  spline S42 degree 5 poles (-30.2612, 78.3022) (-30.274, 78.3344) (-30.3003, 78.3984) (-30.342, 78.4934) (-30.402, 78.618) (-30.4829, 78.771) (-30.568, 78.922) (-30.6557, 79.0719) (-30.7448, 79.221) (-30.8349, 79.3697) (-30.9259, 79.518) (-31.0182, 79.6655) (-31.1123, 79.8122) (-31.2083, 79.9579) (-31.3064, 80.1025) (-31.4063, 80.2462) (-31.5078, 80.389) (-31.6106, 80.5311) (-31.7145, 80.6726) (-31.8195, 80.8135) (-31.9255, 80.9538) (-32.0327, 81.0935) (-32.141, 81.2324) (-32.2506, 81.3707) (-32.3613, 81.5083) (-32.4732, 81.6453) (-32.5861, 81.7816) (-32.7001, 81.9173) (-32.815, 82.0524) (-32.9309, 82.1869) (-33.0477, 82.3208) (-33.1655, 82.4542) (-33.2842, 82.587) (-33.4038, 82.7191) (-33.5244, 82.8507) (-33.6458, 82.9817) (-33.7682, 83.1122) (-33.8914, 83.242) (-34.0154, 83.3714) (-34.1403, 83.5001) (-34.2659, 83.6284) (-34.3924, 83.756) (-34.5197, 83.8832) (-34.6478, 84.0098) (-34.7767, 84.1358) (-34.9063, 84.2613) (-35.0368, 84.3863) (-35.1679, 84.5107) (-35.2998, 84.6346) (-35.4325, 84.758) (-35.5659, 84.8808) (-35.7, 85.0031) (-35.8348, 85.1249) (-35.9703, 85.2462) (-36.1065, 85.367) (-36.2434, 85.4872) (-36.381, 85.607) (-36.5193, 85.7262) (-36.6582, 85.8449) (-36.7978, 85.9631) (-36.938, 86.0807) (-37.0789, 86.1979) (-37.2205, 86.3146) (-37.3627, 86.4307) (-37.5055, 86.5464) (-37.649, 86.6615) (-37.793, 86.7762) (-37.9377, 86.8903) (-38.083, 87.0039) (-38.2289, 87.1171) (-38.3754, 87.2297) (-38.4931, 87.3194) (-38.5816, 87.3865) (-38.6408, 87.4311) (-38.6704, 87.4534) knots 0 0 0 0 0 0 0.01428571 0.02857143 0.04285714 0.05714286 0.07142857 0.08571429 0.1 0.11428571 0.12857143 0.14285714 0.15714286 0.17142857 0.18571429 0.2 0.21428571 0.22857143 0.24285714 0.25714286 0.27142857 0.28571429 0.3 0.31428571 0.32857143 0.34285714 0.35714286 0.37142857 0.38571429 0.4 0.41428571 0.42857143 0.44285714 0.45714286 0.47142857 0.48571429 0.5 0.51428571 0.52857143 0.54285714 0.55714286 0.57142857 0.58571429 0.6 0.61428571 0.62857143 0.64285714 0.65714286 0.67142857 0.68571429 0.7 0.71428571 0.72857143 0.74285714 0.75714286 0.77142857 0.78571429 0.8 0.81428571 0.82857143 0.84285714 0.85714286 0.87142857 0.88571429 0.9 0.91428571 0.92857143 0.94285714 0.95714286 0.97142857 0.98571429 1 1 1 1 1 1
  arc A90 (-38.6704, 87.4534) -> (-42.8523, 85.4395) centre (0.5538, 0.6546) ccw
  spline S43 degree 5 poles (-40.9406, 73.1593) (-40.9578, 73.1893) (-40.9914, 73.2498) (-41.0397, 73.3417) (-41.0997, 73.4662) (-41.1689, 73.6249) (-41.2339, 73.7856) (-41.2964, 73.9476) (-41.3574, 74.1103) (-41.4176, 74.2734) (-41.4767, 74.437) (-41.5345, 74.6011) (-41.5906, 74.7661) (-41.6445, 74.9321) (-41.6965, 75.0989) (-41.7465, 75.2666) (-41.7949, 75.435) (-41.8419, 75.604) (-41.8877, 75.7735) (-41.9324, 75.9434) (-41.976, 76.1138) (-42.0184, 76.2846) (-42.0595, 76.456) (-42.0993, 76.6278) (-42.1379, 76.8002) (-42.1752, 76.973) (-42.2113, 77.1463) (-42.2464, 77.32) (-42.2803, 77.4941) (-42.3133, 77.6686) (-42.3451, 77.8434) (-42.376, 78.0187) (-42.4058, 78.1942) (-42.4345, 78.3702) (-42.4622, 78.5465) (-42.4889, 78.7231) (-42.5146, 78.9001) (-42.5394, 79.0774) (-42.5631, 79.255) (-42.586, 79.4329) (-42.6079, 79.6111) (-42.6288, 79.7896) (-42.6488, 79.9684) (-42.6679, 80.1475) (-42.6861, 80.3268) (-42.7034, 80.5064) (-42.7198, 80.6863) (-42.7353, 80.8664) (-42.7499, 81.0468) (-42.7637, 81.2275) (-42.7766, 81.4083) (-42.7886, 81.5894) (-42.7998, 81.7708) (-42.8101, 81.9523) (-42.8196, 82.1341) (-42.8282, 82.3161) (-42.8361, 82.4984) (-42.8431, 82.6808) (-42.8492, 82.8634) (-42.8546, 83.0462) (-42.8592, 83.2293) (-42.8629, 83.4125) (-42.8659, 83.5959) (-42.868, 83.7795) (-42.8694, 83.9633) (-42.87, 84.1472) (-42.8698, 84.3313) (-42.8688, 84.5156) (-42.8671, 84.7001) (-42.8646, 84.8847) (-42.8613, 85.0694) (-42.8581, 85.2174) (-42.8553, 85.3284) (-42.8533, 85.4025) (-42.8523, 85.4395) knots 0 0 0 0 0 0 0.01428571 0.02857143 0.04285714 0.05714286 0.07142857 0.08571429 0.1 0.11428571 0.12857143 0.14285714 0.15714286 0.17142857 0.18571429 0.2 0.21428571 0.22857143 0.24285714 0.25714286 0.27142857 0.28571429 0.3 0.31428571 0.32857143 0.34285714 0.35714286 0.37142857 0.38571429 0.4 0.41428571 0.42857143 0.44285714 0.45714286 0.47142857 0.48571429 0.5 0.51428571 0.52857143 0.54285714 0.55714286 0.57142857 0.58571429 0.6 0.61428571 0.62857143 0.64285714 0.65714286 0.67142857 0.68571429 0.7 0.71428571 0.72857143 0.74285714 0.75714286 0.77142857 0.78571429 0.8 0.81428571 0.82857143 0.84285714 0.85714286 0.87142857 0.88571429 0.9 0.91428571 0.92857143 0.94285714 0.95714286 0.97142857 0.98571429 1 1 1 1 1 1
  line L43 (-40.9406, 73.1593) -> (-40.1986, 71.8622)
  arc A91 (-40.4866, 70.783) -> (-40.1986, 71.8622) centre (-40.8875, 71.4681) ccw
  arc A92 (-40.4866, 70.783) -> (-44.8229, 68.0584) centre (0.5538, 0.6546) ccw
  arc A93 (-45.9202, 68.2671) -> (-44.8229, 68.0584) centre (-45.2661, 68.7168) ccw
  line L44 (-45.9202, 68.2671) -> (-46.7668, 69.4984)
  spline S44 degree 5 poles (-46.7668, 69.4984) (-46.7864, 69.527) (-46.8263, 69.5835) (-46.8882, 69.6668) (-46.9744, 69.7749) (-47.0872, 69.9061) (-47.2038, 70.0344) (-47.3227, 70.161) (-47.4428, 70.2866) (-47.5636, 70.4116) (-47.6854, 70.5358) (-47.8082, 70.6591) (-47.9325, 70.7812) (-48.0586, 70.9018) (-48.1864, 71.021) (-48.3158, 71.1388) (-48.4465, 71.2555) (-48.5784, 71.3712) (-48.7112, 71.486) (-48.8449, 71.6) (-48.9795, 71.7132) (-49.115, 71.8255) (-49.2516, 71.9369) (-49.3891, 72.0473) (-49.5277, 72.1569) (-49.6672, 72.2655) (-49.8077, 72.3732) (-49.949, 72.4802) (-50.0911, 72.5863) (-50.234, 72.6917) (-50.3777, 72.7962) (-50.5222, 72.9) (-50.6674, 73.0031) (-50.8135, 73.1053) (-50.9603, 73.2068) (-51.1079, 73.3075) (-51.2562, 73.4074) (-51.4052, 73.5066) (-51.5549, 73.6051) (-51.7053, 73.7029) (-51.8563, 73.7999) (-52.0081, 73.8962) (-52.1604, 73.9919) (-52.3135, 74.0868) (-52.4672, 74.181) (-52.6215, 74.2745) (-52.7765, 74.3673) (-52.932, 74.4594) (-53.0882, 74.5508) (-53.245, 74.6416) (-53.4024, 74.7317) (-53.5603, 74.8211) (-53.7188, 74.9099) (-53.878, 74.998) (-54.0376, 75.0854) (-54.1978, 75.1721) (-54.3586, 75.2583) (-54.5199, 75.3437) (-54.6818, 75.4285) (-54.8442, 75.5127) (-55.0071, 75.5962) (-55.1706, 75.6791) (-55.3345, 75.7613) (-55.499, 75.8429) (-55.664, 75.9239) (-55.8295, 76.0042) (-55.9954, 76.0839) (-56.1619, 76.163) (-56.3288, 76.2415) (-56.4962, 76.3193) (-56.6641, 76.3965) (-56.7988, 76.4578) (-56.9001, 76.5035) (-56.9677, 76.5338) (-57.0015, 76.549) knots 0 0 0 0 0 0 0.01428571 0.02857143 0.04285714 0.05714286 0.07142857 0.08571429 0.1 0.11428571 0.12857143 0.14285714 0.15714286 0.17142857 0.18571429 0.2 0.21428571 0.22857143 0.24285714 0.25714286 0.27142857 0.28571429 0.3 0.31428571 0.32857143 0.34285714 0.35714286 0.37142857 0.38571429 0.4 0.41428571 0.42857143 0.44285714 0.45714286 0.47142857 0.48571429 0.5 0.51428571 0.52857143 0.54285714 0.55714286 0.57142857 0.58571429 0.6 0.61428571 0.62857143 0.64285714 0.65714286 0.67142857 0.68571429 0.7 0.71428571 0.72857143 0.74285714 0.75714286 0.77142857 0.78571429 0.8 0.81428571 0.82857143 0.84285714 0.85714286 0.87142857 0.88571429 0.9 0.91428571 0.92857143 0.94285714 0.95714286 0.97142857 0.98571429 1 1 1 1 1 1
  arc A94 (-57.0015, 76.549) -> (-60.6304, 73.655) centre (0.5538, 0.6546) ccw
  spline S45 degree 5 poles (-56.034, 62.108) (-56.0575, 62.1335) (-56.1038, 62.185) (-56.1712, 62.2638) (-56.2574, 62.3719) (-56.3602, 62.5112) (-56.4594, 62.6534) (-56.5563, 62.7974) (-56.6521, 62.9424) (-56.747, 63.0881) (-56.841, 63.2344) (-56.9339, 63.3816) (-57.0253, 63.53) (-57.1148, 63.6797) (-57.2026, 63.8309) (-57.2886, 63.9832) (-57.3733, 64.1366) (-57.4567, 64.2909) (-57.5391, 64.4459) (-57.6205, 64.6017) (-57.7009, 64.7581) (-57.7803, 64.9152) (-57.8585, 65.0731) (-57.9355, 65.2318) (-58.0115, 65.3913) (-58.0863, 65.5515) (-58.1601, 65.7124) (-58.2329, 65.8739) (-58.3048, 66.0361) (-58.3757, 66.1989) (-58.4457, 66.3622) (-58.5147, 66.5262) (-58.5829, 66.6907) (-58.65, 66.8559) (-58.7163, 67.0216) (-58.7816, 67.1879) (-58.8461, 67.3547) (-58.9096, 67.522) (-58.9723, 67.6899) (-59.0342, 67.8583) (-59.0952, 68.0271) (-59.1553, 68.1965) (-59.2146, 68.3663) (-59.2731, 68.5367) (-59.3307, 68.7075) (-59.3876, 68.8787) (-59.4436, 69.0505) (-59.4988, 69.2226) (-59.5532, 69.3952) (-59.6068, 69.5683) (-59.6596, 69.7417) (-59.7116, 69.9156) (-59.7628, 70.0899) (-59.8133, 70.2647) (-59.863, 70.4398) (-59.912, 70.6153) (-59.9601, 70.7912) (-60.0075, 70.9675) (-60.0542, 71.1442) (-60.1001, 71.3212) (-60.1453, 71.4986) (-60.1897, 71.6764) (-60.2334, 71.8546) (-60.2764, 72.0331) (-60.3186, 72.212) (-60.3601, 72.3912) (-60.4009, 72.5707) (-60.441, 72.7506) (-60.4803, 72.9308) (-60.5189, 73.1113) (-60.5569, 73.2922) (-60.5866, 73.4372) (-60.6086, 73.546) (-60.6232, 73.6187) (-60.6304, 73.655) knots 0 0 0 0 0 0 0.01428571 0.02857143 0.04285714 0.05714286 0.07142857 0.08571429 0.1 0.11428571 0.12857143 0.14285714 0.15714286 0.17142857 0.18571429 0.2 0.21428571 0.22857143 0.24285714 0.25714286 0.27142857 0.28571429 0.3 0.31428571 0.32857143 0.34285714 0.35714286 0.37142857 0.38571429 0.4 0.41428571 0.42857143 0.44285714 0.45714286 0.47142857 0.48571429 0.5 0.51428571 0.52857143 0.54285714 0.55714286 0.57142857 0.58571429 0.6 0.61428571 0.62857143 0.64285714 0.65714286 0.67142857 0.68571429 0.7 0.71428571 0.72857143 0.74285714 0.75714286 0.77142857 0.78571429 0.8 0.81428571 0.82857143 0.84285714 0.85714286 0.87142857 0.88571429 0.9 0.91428571 0.92857143 0.94285714 0.95714286 0.97142857 0.98571429 1 1 1 1 1 1
  line L45 (-56.034, 62.108) -> (-55.022, 61.0086)
  arc A95 (-55.0627, 59.8924) -> (-55.022, 61.0086) centre (-55.606, 60.4711) ccw
  arc A96 (-55.0627, 59.8924) -> (-58.6839, 56.2712) centre (0.5538, 0.6546) ccw
  arc A97 (-59.8002, 56.2305) -> (-58.6839, 56.2712) centre (-59.2626, 56.8145) ccw
  line L46 (-59.8002, 56.2305) -> (-60.8996, 57.2425)
  spline S46 degree 5 poles (-60.8996, 57.2425) (-60.925, 57.266) (-60.9765, 57.3122) (-61.0553, 57.3797) (-61.1634, 57.4659) (-61.3027, 57.5687) (-61.4449, 57.6679) (-61.5889, 57.7648) (-61.7339, 57.8605) (-61.8796, 57.9555) (-62.0259, 58.0495) (-62.1731, 58.1424) (-62.3215, 58.2337) (-62.4713, 58.3233) (-62.6224, 58.411) (-62.7747, 58.4971) (-62.9282, 58.5818) (-63.0824, 58.6652) (-63.2375, 58.7476) (-63.3932, 58.829) (-63.5496, 58.9094) (-63.7067, 58.9887) (-63.8646, 59.067) (-64.0233, 59.144) (-64.1828, 59.22) (-64.343, 59.2948) (-64.5039, 59.3686) (-64.6655, 59.4414) (-64.8276, 59.5133) (-64.9904, 59.5842) (-65.1538, 59.6542) (-65.3177, 59.7232) (-65.4823, 59.7913) (-65.6474, 59.8585) (-65.8131, 59.9248) (-65.9794, 59.9901) (-66.1462, 60.0545) (-66.3135, 60.1181) (-66.4814, 60.1808) (-66.6498, 60.2427) (-66.8186, 60.3037) (-66.988, 60.3638) (-67.1579, 60.4231) (-67.3282, 60.4816) (-67.499, 60.5392) (-67.6703, 60.596) (-67.842, 60.652) (-68.0141, 60.7072) (-68.1868, 60.7616) (-68.3598, 60.8152) (-68.5333, 60.8681) (-68.7072, 60.9201) (-68.8815, 60.9713) (-69.0562, 61.0218) (-69.2313, 61.0715) (-69.4068, 61.1204) (-69.5827, 61.1686) (-69.759, 61.216) (-69.9357, 61.2627) (-70.1127, 61.3086) (-70.2902, 61.3538) (-70.468, 61.3982) (-70.6461, 61.4419) (-70.8246, 61.4849) (-71.0035, 61.5271) (-71.1827, 61.5686) (-71.3622, 61.6094) (-71.5421, 61.6494) (-71.7223, 61.6888) (-71.9029, 61.7274) (-72.0837, 61.7653) (-72.2287, 61.7951) (-72.3375, 61.8171) (-72.4102, 61.8316) (-72.4465, 61.8389) knots 0 0 0 0 0 0 0.01428571 0.02857143 0.04285714 0.05714286 0.07142857 0.08571429 0.1 0.11428571 0.12857143 0.14285714 0.15714286 0.17142857 0.18571429 0.2 0.21428571 0.22857143 0.24285714 0.25714286 0.27142857 0.28571429 0.3 0.31428571 0.32857143 0.34285714 0.35714286 0.37142857 0.38571429 0.4 0.41428571 0.42857143 0.44285714 0.45714286 0.47142857 0.48571429 0.5 0.51428571 0.52857143 0.54285714 0.55714286 0.57142857 0.58571429 0.6 0.61428571 0.62857143 0.64285714 0.65714286 0.67142857 0.68571429 0.7 0.71428571 0.72857143 0.74285714 0.75714286 0.77142857 0.78571429 0.8 0.81428571 0.82857143 0.84285714 0.85714286 0.87142857 0.88571429 0.9 0.91428571 0.92857143 0.94285714 0.95714286 0.97142857 0.98571429 1 1 1 1 1 1
  arc A98 (-72.4465, 61.8389) -> (-75.3405, 58.21) centre (0.5538, 0.6546) ccw
  spline S47 degree 5 poles (-68.2899, 47.9753) (-68.3185, 47.9949) (-68.375, 48.0348) (-68.4583, 48.0966) (-68.5664, 48.1828) (-68.6976, 48.2957) (-68.826, 48.4123) (-68.9525, 48.5312) (-69.0781, 48.6512) (-69.2031, 48.7721) (-69.3273, 48.8938) (-69.4506, 49.0167) (-69.5727, 49.141) (-69.6933, 49.2671) (-69.8125, 49.3949) (-69.9303, 49.5243) (-70.047, 49.655) (-70.1627, 49.7869) (-70.2775, 49.9197) (-70.3915, 50.0534) (-70.5047, 50.1879) (-70.617, 50.3235) (-70.7284, 50.46) (-70.8389, 50.5976) (-70.9484, 50.7362) (-71.057, 50.8757) (-71.1647, 51.0162) (-71.2717, 51.1575) (-71.3778, 51.2996) (-71.4832, 51.4425) (-71.5878, 51.5862) (-71.6916, 51.7307) (-71.7946, 51.8759) (-71.8968, 52.022) (-71.9983, 52.1688) (-72.099, 52.3164) (-72.1989, 52.4646) (-72.2982, 52.6136) (-72.3966, 52.7633) (-72.4944, 52.9137) (-72.5914, 53.0648) (-72.6878, 53.2165) (-72.7834, 53.3689) (-72.8783, 53.522) (-72.9725, 53.6757) (-73.066, 53.83) (-73.1588, 53.9849) (-73.2509, 54.1405) (-73.3424, 54.2967) (-73.4331, 54.4535) (-73.5232, 54.6108) (-73.6126, 54.7688) (-73.7014, 54.9273) (-73.7895, 55.0864) (-73.8769, 55.2461) (-73.9637, 55.4063) (-74.0498, 55.5671) (-74.1352, 55.7284) (-74.22, 55.8903) (-74.3042, 56.0527) (-74.3877, 56.2156) (-74.4706, 56.3791) (-74.5528, 56.543) (-74.6344, 56.7075) (-74.7154, 56.8725) (-74.7958, 57.0379) (-74.8755, 57.2039) (-74.9545, 57.3704) (-75.033, 57.5373) (-75.1108, 57.7047) (-75.1881, 57.8726) (-75.2493, 58.0073) (-75.295, 58.1086) (-75.3253, 58.1761) (-75.3405, 58.21) knots 0 0 0 0 0 0 0.01428571 0.02857143 0.04285714 0.05714286 0.07142857 0.08571429 0.1 0.11428571 0.12857143 0.14285714 0.15714286 0.17142857 0.18571429 0.2 0.21428571 0.22857143 0.24285714 0.25714286 0.27142857 0.28571429 0.3 0.31428571 0.32857143 0.34285714 0.35714286 0.37142857 0.38571429 0.4 0.41428571 0.42857143 0.44285714 0.45714286 0.47142857 0.48571429 0.5 0.51428571 0.52857143 0.54285714 0.55714286 0.57142857 0.58571429 0.6 0.61428571 0.62857143 0.64285714 0.65714286 0.67142857 0.68571429 0.7 0.71428571 0.72857143 0.74285714 0.75714286 0.77142857 0.78571429 0.8 0.81428571 0.82857143 0.84285714 0.85714286 0.87142857 0.88571429 0.9 0.91428571 0.92857143 0.94285714 0.95714286 0.97142857 0.98571429 1 1 1 1 1 1
  line L47 (-68.2899, 47.9753) -> (-67.0586, 47.1287)
  arc A99 (-66.8499, 46.0313) -> (-67.0586, 47.1287) centre (-67.5084, 46.4746) ccw
  arc A100 (-66.8499, 46.0313) -> (-69.5745, 41.6951) centre (0.5538, 0.6546) ccw
  arc A101 (-70.6538, 41.4071) -> (-69.5745, 41.6951) centre (-70.2596, 42.096) ccw
  line L48 (-70.6538, 41.4071) -> (-71.9508, 42.1491)